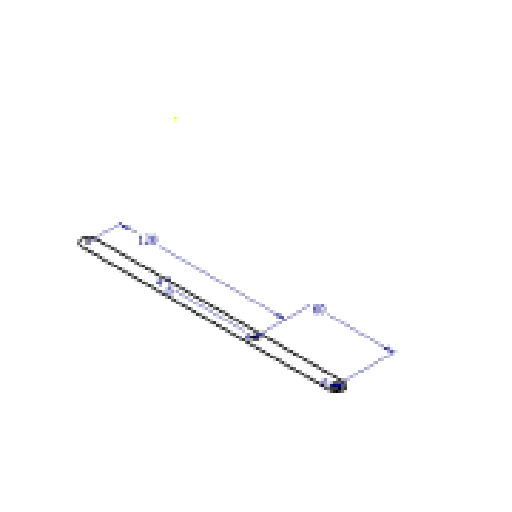
# Autodesk Inventor part: Guides
Saved by Autodesk Inventor 2023 (Build 270158000, 158)
## iProperties
Created: 2022-11-08
Part Number: Guides
Material: Generic
Document SubType Name: Modeling
Designer: deli
Density: 1 g/cm^3
Appearance: Default
Author: deli
Autodesk Inventor part; units mm, degrees
ref_plane "YZ Plane" through (0, 0, 0) normal (1, 0, 0) x (0, 1, 0)
ref_plane "XZ Plane" through (0, 0, 0) normal (0, 1, 0) x (-1, 0, 0)
ref_plane "XY Plane" through (0, 0, 0) normal (0, 0, 1) x (1, 0, 0)
sketch "Sketch1" plane through (0, 0, 0) normal (0, 1, 0) x (-1, 0, 0)
  circle A0 centre (-166.0092, 108.4393) radius 2
  line L0 (-46.0092, 114.4393) -> (-226.0092, 114.4393)
  line L1 (-46.0092, 104.4393) -> (-226.0092, 104.4393)
  arc A1 (-46.0092, 104.4393) -> (-46.0092, 114.4393) centre (-46.0092, 109.4393) ccw
  arc A2 (-226.0092, 114.4393) -> (-226.0092, 104.4393) centre (-226.0092, 109.4393) ccw
  circle A3 centre (-226.0092, 109.4393) radius 3
  point P0 (0, 0)
  dimension "d0" = 4
  dimension "d2" = 4
  dimension "d3" = 6
  dimension "d4" = 6
  dimension "d5" = 60
  dimension "d6" = 120
  constraints: 4 centre point, 4 end point, 4 point on circle, 4 tangent, 2 horizontal, 1 coincident
  measures "d0" diameter of A0
  measures "d2" distance from line of L1 A0.centre
  measures "d3" distance from line of L0 A0.centre
  measures "d4" diameter of A3
  measures "d5" horizontal distance of A0.centre A3.centre
  measures "d6" horizontal distance of A1.centre A0.centre
extrude "Extrusion1" add sketch "Sketch1" along normal blind 3.175
body "Solid1"
